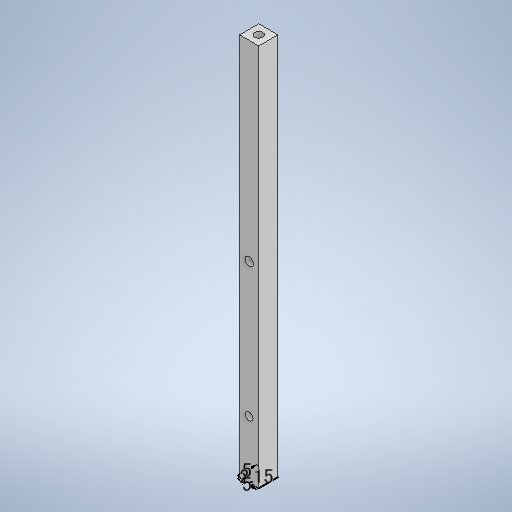
# Autodesk Inventor part: g_a_exp
Saved by Autodesk Inventor 2025 (Build 290162000, 162)
## iProperties
Created: 2024-07-31
Part Number: g_a_exp
Material: 一般
Document SubType Name: Modeling
Designer: Saigusa
Density: 1 g/cm^3
Appearance: 既定
Author: Saigusa
Autodesk Inventor part; units mm, degrees
ref_plane "YZ Plane" through (0, 0, 0) normal (1, 0, 0) x (0, 1, 0)
ref_plane "XZ Plane" through (0, 0, 0) normal (0, 1, 0) x (-1, 0, 0)
ref_plane "XY Plane" through (0, 0, 0) normal (0, 0, 1) x (1, 0, 0)
sketch "スケッチ1" plane through (0, 0, 0) normal (0, 1, 0) x (-1, 0, 0)
  circle A0 centre (0, 0) radius 1.075
  line L0 (-2.5, -2.5) -> (2.5, -2.5)
  line L1 (2.5, -2.5) -> (2.5, 2.5)
  line L2 (2.5, 2.5) -> (-2.5, 2.5)
  line L3 (-2.5, 2.5) -> (-2.5, -2.5)
  line L4 (-2.5, -2.5) -> (2.5, 2.5) construction
  line L5 (2.5, -2.5) -> (-2.5, 2.5) construction
  dimension "d0" = 2.15
  dimension "d1" = 5
  dimension "d2" = 5
  constraints: 12 end point, 2 midpoint, 2 parallel, 1 centre point, 1 coincident, 1 horizontal, 1 perpendicular
  measures "d0" diameter of A0
  measures "d1" distance of L2.end L1.end
  measures "d2" distance of L1.end L0.end
extrude "押し出し1" add sketch "スケッチ1" along normal blind 100 contours A0 | L3 L2 L1 L0
extrude "押し出し2" cut sketch "スケッチ1" along normal blind 15 contours A0
sketch "スケッチ2" plane through (0, 100, 0) normal (0, 1, 0) x (1, 0, 0)
  point P0 (0, 0)
hole "穴1" at (0, 100, 0) direction (0, -1, 0) diameter 2.15 depth 50 tip angle 118
sketch "スケッチ3" plane through (2.5, 0, -2.5) normal (0, 0, -1) x (-1, 0, 0)
  line L0 (5, 0) -> (0, 0) projected
  line L1 (5, 0) -> (5, 100) projected
  line L2 (0, 0) -> (5, 0)
  line L3 (5, 0) -> (5, 15)
  line L4 (5, 15) -> (0, 15)
  line L5 (0, 15) -> (0, 0)
  circle A0 centre (2.5, 15) radius 1
  line L6 (0, 100) -> (5, 100) projected
  line L7 (0, 100) -> (5, 100)
  line L8 (5, 100) -> (5, 50)
  line L9 (5, 50) -> (0, 50)
  line L10 (0, 50) -> (0, 100)
  circle A1 centre (2.5, 50) radius 1.1
  point P0 (2.5, 0)
  dimension "d14" = 15
  dimension "d15" = 2
  dimension "d16" = 50
  dimension "d17" = 2.2
  constraints: 16 end point, 4 parallel, 3 midpoint, 2 centre point, 2 horizontal, 2 perpendicular, 1 point on line
  measures "d14" distance of L3.end L2.end
  measures "d15" diameter of A0
  measures "d16" distance of L7.end L8.end
  measures "d17" diameter of A1
extrude "押し出し3" cut sketch "スケッチ3" against normal blind 5 contours A0 L4 | L4 A0 | A1 L9 | L9 A1
